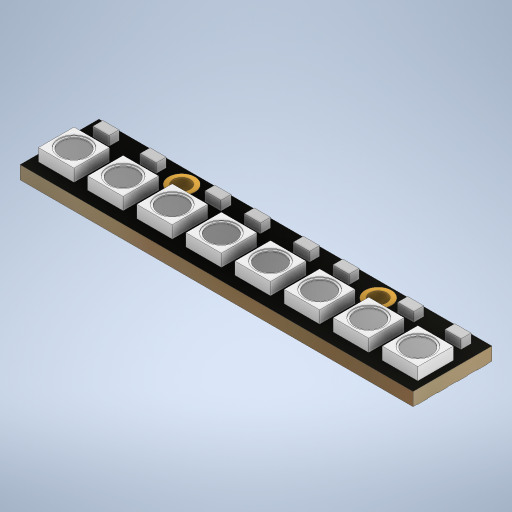
# Autodesk Inventor part: LED
Saved by Autodesk Inventor 2023 (Build 270158000, 158)
## iProperties
Created: 2023-03-17
Part Number: LED
Material: Generic
Document SubType Name: Modeling
Designer: Amos Yu
Density: 1 g/cm^3
Appearance: Default
Author: Amos Yu
Autodesk Inventor part; units mm, degrees
ref_plane "YZ Plane" through (0, 0, 0) normal (1, 0, 0) x (0, 1, 0)
sketch "Sketch1" plane through (0, 0, 0) normal (0, 1, 0) x (-1, 0, 0)
  line L0 (0, 0) -> (50.8, 0)
  line L1 (50.8, 0) -> (50.8, -10.2)
  line L2 (50.8, -10.2) -> (0, -10.2)
  line L3 (0, -10.2) -> (0, 0)
  dimension "d0" = 50.8
  dimension "d1" = 10.2
  constraints: 8 end point, 2 parallel, 1 horizontal, 1 perpendicular
  measures "d0" distance of L1.end L2.end
  measures "d1" distance of L2.end L0.start
extrude "Extrusion1" add sketch "Sketch1" along normal blind 1.7
sketch "Sketch2" plane through (0, 0, 0) normal (0, -1, 0) x (1, 0, 0)
  line L0 (-5.475, -1.5) -> (-0.875, -1.5)
  line L1 (-0.875, -1.5) -> (-0.875, -6.1)
  line L2 (-0.875, -6.1) -> (-5.475, -6.1)
  line L3 (-5.475, -6.1) -> (-5.475, -1.5)
  line L4 (0, 0) -> (0, -10.2) projected
  line L5 (-50.8, 0) -> (0, 0) projected
  line L6 (-11.825, -1.5) -> (-7.225, -1.5)
  line L7 (-7.225, -1.5) -> (-7.225, -6.1)
  line L8 (-7.225, -6.1) -> (-11.825, -6.1)
  line L9 (-11.825, -6.1) -> (-11.825, -1.5)
  line L10 (-18.175, -1.5) -> (-13.575, -1.5)
  line L11 (-13.575, -1.5) -> (-13.575, -6.1)
  line L12 (-13.575, -6.1) -> (-18.175, -6.1)
  line L13 (-18.175, -6.1) -> (-18.175, -1.5)
  line L14 (-24.525, -1.5) -> (-19.925, -1.5)
  line L15 (-19.925, -1.5) -> (-19.925, -6.1)
  line L16 (-19.925, -6.1) -> (-24.525, -6.1)
  line L17 (-24.525, -6.1) -> (-24.525, -1.5)
  line L18 (-30.875, -1.5) -> (-26.275, -1.5)
  line L19 (-26.275, -1.5) -> (-26.275, -6.1)
  line L20 (-26.275, -6.1) -> (-30.875, -6.1)
  line L21 (-30.875, -6.1) -> (-30.875, -1.5)
  line L22 (-37.225, -1.5) -> (-32.625, -1.5)
  line L23 (-32.625, -1.5) -> (-32.625, -6.1)
  line L24 (-32.625, -6.1) -> (-37.225, -6.1)
  line L25 (-37.225, -6.1) -> (-37.225, -1.5)
  line L26 (-43.575, -1.5) -> (-38.975, -1.5)
  line L27 (-38.975, -1.5) -> (-38.975, -6.1)
  line L28 (-38.975, -6.1) -> (-43.575, -6.1)
  line L29 (-43.575, -6.1) -> (-43.575, -1.5)
  line L30 (-49.925, -1.5) -> (-45.325, -1.5)
  line L31 (-45.325, -1.5) -> (-45.325, -6.1)
  line L32 (-45.325, -6.1) -> (-49.925, -6.1)
  line L33 (-49.925, -6.1) -> (-49.925, -1.5)
  dimension "d4" = 4.6
  dimension "d5" = 4.6
  dimension "d6" = 0.875
  dimension "d7" = 1.5
  dimension "d10" = 6.35
  constraints: 64 end point, 2 horizontal, 2 parallel, 1 perpendicular, 56 other
  measures "d4" distance of L1.end L2.end
  measures "d5" distance of L0.end L1.end
  measures "d6" distance between parallel lines of L4 L1
  measures "d7" distance between parallel lines of L5 L0
  measures "d10" distance of L0.start L6.start
extrude "Extrusion2" add sketch "Sketch2" against normal blind 3.3
sketch "Sketch3" plane through (0, 3.3, 0) normal (0, 1, 0) x (1, 0, 0)
  line L0 (-5.475, 6.1) -> (-5.475, 1.5) projected
  line L1 (-0.875, 6.1) -> (-5.475, 6.1) projected
  circle A0 centre (-3.175, 3.8) radius 2
  circle A1 centre (-3.175, 3.8) radius 1.75
  circle A2 centre (-9.525, 3.8) radius 2
  circle A3 centre (-9.525, 3.8) radius 1.75
  circle A4 centre (-15.875, 3.8) radius 2
  circle A5 centre (-15.875, 3.8) radius 1.75
  circle A6 centre (-22.225, 3.8) radius 2
  circle A7 centre (-22.225, 3.8) radius 1.75
  circle A8 centre (-28.575, 3.8) radius 2
  circle A9 centre (-28.575, 3.8) radius 1.75
  circle A10 centre (-34.925, 3.8) radius 2
  circle A11 centre (-34.925, 3.8) radius 1.75
  circle A12 centre (-41.275, 3.8) radius 2
  circle A13 centre (-41.275, 3.8) radius 1.75
  circle A14 centre (-47.625, 3.8) radius 2
  circle A15 centre (-47.625, 3.8) radius 1.75
  point P0 (0, 0)
  point P1 (-3.175, 6.1)
  point P2 (-5.475, 3.8)
  dimension "d17" = 4
  dimension "d18" = 3.5
  dimension "d21" = 6.35
  constraints: 16 centre point, 8 coincident, 2 midpoint, 1 horizontal, 1 horizontal alignment, 1 vertical alignment, 28 other
  measures "d17" diameter of A0
  measures "d18" diameter of A1
  measures "d21" distance of A0.centre A2.centre
extrude "Extrusion3" cut sketch "Sketch3" against normal blind 0.2 contours A1 | A3 | A5 | A7 | A9 | A11 | A13 | A15
extrude "Extrusion4" cut sketch "Sketch3" against normal blind 0.1 contours A0 | A1 | A2 | A3 | A4 | A5 | A6 | A7 | A8 | A9 | A10 | A11 | A12 | A13 | A14 | A15
sketch "Sketch4" plane through (0, 1.7, 0) normal (0, 1, 0) x (1, 0, 0)
  line L0 (0, 0) -> (0, 10.2) projected
  line L1 (-50.8, 10.2) -> (-50.8, 0) projected
  line L2 (0, 10.2) -> (-50.8, 10.2) projected
  point P0 (-38.1, 8.2)
  point P1 (-12.7, 8.2)
  dimension "d37" = 12.7
  dimension "d39" = 12.7
  dimension "d40" = 2
  constraints: 1 horizontal alignment
  measures "d37" distance from line of L0 point (-12.7, 8.2)
  measures "d39" distance from line of L1 point (-38.1, 8.2)
  measures "d40" distance from line of L2 point (-12.7, 8.2)
hole "Hole1" at (-38.1, 1.7, -8.2) at (-12.7, 1.7, -8.2) direction (0, -1, 0) diameter 2.2 end through all
sketch "Sketch5" plane through (0, 1.7, 0) normal (0, 1, 0) x (1, 0, 0)
  line L0 (-3.7, 7.8) -> (-1.6, 7.8)
  line L1 (-1.6, 7.8) -> (-1.6, 9.1)
  line L2 (-1.6, 9.1) -> (-3.7, 9.1)
  line L3 (-3.7, 9.1) -> (-3.7, 7.8)
  line L4 (0, 0) -> (0, 10.2) projected
  line L5 (0, 10.2) -> (-50.8, 10.2) projected
  line L6 (-9.8, 7.8) -> (-7.7, 7.8)
  line L7 (-7.7, 7.8) -> (-7.7, 9.1)
  line L8 (-7.7, 9.1) -> (-9.8, 9.1)
  line L9 (-9.8, 9.1) -> (-9.8, 7.8)
  line L10 (-18.175, 7.8) -> (-16.075, 7.8)
  line L11 (-16.075, 7.8) -> (-16.075, 9.1)
  line L12 (-16.075, 9.1) -> (-18.175, 9.1)
  line L13 (-18.175, 9.1) -> (-18.175, 7.8)
  line L14 (-23.275, 7.8) -> (-21.175, 7.8)
  line L15 (-21.175, 7.8) -> (-21.175, 9.1)
  line L16 (-21.175, 9.1) -> (-23.275, 9.1)
  line L17 (-23.275, 9.1) -> (-23.275, 7.8)
  line L18 (-19.925, 6.1) -> (-24.525, 6.1) projected
  point P0 (-7.7, 8.45)
  point P1 (-18.175, 6.1)
  point P2 (-22.225, 7.8)
  point P3 (-22.225, 6.1)
  dimension "d41" = 2.1
  dimension "d42" = 1.3
  dimension "d43" = 3.7
  dimension "d44" = 2.4
  dimension "d45" = 2.1
  dimension "d46" = 1.3
  dimension "d47" = 2.1
  dimension "d48" = 1.3
  dimension "d49" = 2.1
  dimension "d50" = 1.3
  dimension "d51" = 4
  constraints: 32 end point, 8 parallel, 4 horizontal, 4 perpendicular, 3 horizontal alignment, 3 midpoint, 2 vertical alignment
  measures "d41" distance of L2.end L1.end
  measures "d42" distance of L1.end L0.end
  measures "d43" distance between parallel lines of L4 L3
  measures "d44" distance between parallel lines of L5 L0
  measures "d45" distance of L8.end L7.end
  measures "d46" distance of L7.end L6.end
  measures "d47" distance of L12.end L11.end
  measures "d48" distance of L11.end L10.end
  measures "d49" distance of L16.end L15.end
  measures "d50" distance of L15.end L14.end
  measures "d51" distance from line of point (-7.7, 8.45) L3
extrude "Extrusion5" add sketch "Sketch5" along normal blind 1.2
ref_plane "Work Plane1" through (-25.4, 0, 0) normal (1, 0, 0) x (0, 0, -1)
sketch "Sketch6" plane through (0, 0, 0) normal (0, -1, 0) x (1, 0, 0)
  line L0 (0, -9.575) -> (-2.5, -9.575)
  line L1 (-2.5, -9.575) -> (-2.5, -8.275)
  line L2 (-2.5, -8.275) -> (0, -8.275)
  line L3 (0, -8.275) -> (0, -9.575)
  line L4 (0, -7.025) -> (-2.5, -7.025)
  line L5 (-2.5, -7.025) -> (-2.5, -5.725)
  line L6 (-2.5, -5.725) -> (0, -5.725)
  line L7 (0, -5.725) -> (0, -7.025)
  line L8 (0, -4.475) -> (-2.5, -4.475)
  line L9 (-2.5, -4.475) -> (-2.5, -3.175)
  line L10 (-2.5, -3.175) -> (0, -3.175)
  line L11 (0, -3.175) -> (0, -4.475)
  line L12 (0, -1.925) -> (-2.5, -1.925)
  line L13 (-2.5, -1.925) -> (-2.5, -0.625)
  line L14 (-2.5, -0.625) -> (0, -0.625)
  line L15 (0, -0.625) -> (0, -1.925)
  line L16 (0, -10.2) -> (-50.8, -10.2) projected
  line L17 (0, 0) -> (0, -10.2) projected
  circle A0 centre (-12.7, -8.2) radius 1.1 projected
  circle A1 centre (-12.7, -8.2) radius 1.1 projected
  circle A2 centre (-12.7, -8.2) radius 1.7
  dimension "d54" = 2.5
  dimension "d55" = 1.3
  dimension "d58" = 2.55
  dimension "d63" = 0.625
  dimension "d64" = 3.4
  constraints: 32 end point, 2 collinear, 2 parallel, 1 centre point, 1 coincident, 1 horizontal, 1 perpendicular, 1 vertical, 23 other
  measures "d54" distance of L1.end L2.end
  measures "d55" distance of L0.end L1.end
  measures "d58" distance of L0.start L4.start
  measures "d63" distance between parallel lines of L16 L0
  measures "d64" diameter of A2
extrude "Extrusion6" add sketch "Sketch6" along normal blind 0.05
sketch "Sketch7" plane through (0, 1.7, 0) normal (0, 1, 0) x (1, 0, 0)
  circle A0 centre (-12.7, 8.2) radius 1.1 projected
  circle A1 centre (-12.7, 8.2) radius 1.7
  point P0 (0, 0)
  dimension "d67" = 3.4
  constraints: 1 centre point, 1 coincident
  measures "d67" diameter of A1
extrude "Extrusion7" add sketch "Sketch7" along normal blind 0.05
mirror "Mirror1" about plane through (-25.4, 0, 0) normal (1, 0, 0) of "Extrusion7", "Extrusion5", "Extrusion6"
ref_plane "Work Plane2" through (0, 0, -5.1) normal (0, 0, -1) x (-1, 0, 0)
body "Solid1"
